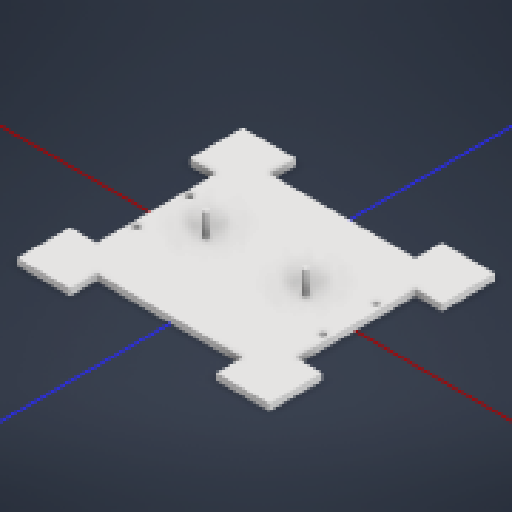
# Autodesk Inventor part: base
Saved by Autodesk Inventor 2025.4 (Build 294407000, 407)
## iProperties
Created: 2026-09-12
Part Number: base
Material: Generic
Document SubType Name: Modeling
Designer: User
Density: 1 g/cm^3
Appearance: Default
Author: User
Autodesk Inventor part; units mm, degrees
ref_plane "YZ Plane" through (0, 0, 0) normal (1, 0, 0) x (0, 1, 0)
ref_plane "XZ Plane" through (0, 0, 0) normal (0, 1, 0) x (-1, 0, 0)
ref_plane "XY Plane" through (0, 0, 0) normal (0, 0, 1) x (1, 0, 0)
sketch "Sketch1" plane through (0, 0, 0) normal (0, 1, 0) x (-1, 0, 0)
  line L0 (15, 13) -> (-15, 13)
  line L1 (-15, 13) -> (-15, -13)
  line L2 (-15, -13) -> (15, -13)
  line L3 (15, -13) -> (15, 13)
  line L4 (15, 13) -> (-15, -13) construction
  line L5 (-15, 13) -> (15, -13) construction
  circle A0 centre (-14, 4) radius 0.5
  circle A1 centre (14, 4) radius 0.5
  circle A2 centre (14, -4) radius 0.5
  circle A3 centre (-14, -4) radius 0.5
  line L6 (-11, 17) -> (-19, 17)
  line L7 (-19, 17) -> (-19, 9)
  line L8 (-19, 9) -> (-11, 9)
  line L9 (-11, 9) -> (-11, 17)
  line L10 (-11, 17) -> (-19, 9) construction
  line L11 (-19, 17) -> (-11, 9) construction
  line L12 (19, 9) -> (11, 9)
  line L13 (11, 9) -> (11, 17)
  line L14 (11, 17) -> (19, 17)
  line L15 (19, 17) -> (19, 9)
  line L16 (19, 9) -> (11, 17) construction
  line L17 (11, 9) -> (19, 17) construction
  line L18 (19, -17) -> (11, -17)
  line L19 (11, -17) -> (11, -9)
  line L20 (11, -9) -> (19, -9)
  line L21 (19, -9) -> (19, -17)
  line L22 (19, -17) -> (11, -9) construction
  line L23 (11, -17) -> (19, -9) construction
  line L24 (-11, -9) -> (-19, -9)
  line L25 (-19, -9) -> (-19, -17)
  line L26 (-19, -17) -> (-11, -17)
  line L27 (-11, -17) -> (-11, -9)
  line L28 (-11, -9) -> (-19, -17) construction
  line L29 (-19, -9) -> (-11, -17) construction
  point P0 (0, 0)
  point P1 (11, 13)
  point P2 (15, 9)
  point P3 (15, -9)
  point P4 (11, -13)
  point P5 (-11, -13)
  point P6 (-15, -9)
  point P7 (-15, 9)
  point P8 (-11, 13)
  dimension "d0" = 30
  dimension "d1" = 26
  dimension "d4" = 1
  dimension "d5" = 9
  dimension "d6" = 1
  dimension "d7" = 1
  dimension "d8" = 1
  dimension "d9" = 1
  dimension "d10" = 1
  dimension "d11" = 9
  dimension "d12" = 1
  dimension "d13" = 9
  dimension "d14" = 9
  dimension "d15" = 1
  dimension "d24" = 8
  dimension "d25" = 8
  dimension "d26" = 8
  dimension "d27" = 8
  dimension "d28" = 8
  dimension "d29" = 8
  dimension "d30" = 8
  dimension "d31" = 8
  constraints: 60 end point, 10 midpoint, 10 parallel, 5 horizontal, 5 perpendicular, 4 centre point
  measures "d0" distance of L2.end L1.end
  measures "d1" distance of L1.end L0.end
  measures "d4" diameter of A0
  measures "d5" distance from line of L0 A0.centre
  measures "d6" distance from line of L1 A0.centre
  measures "d7" diameter of A1
  measures "d8" diameter of A2
  measures "d9" diameter of A3
  measures "d10" distance from line of L1 A3.centre
  measures "d11" distance from line of L2 A3.centre
  measures "d12" distance from line of L3 A2.centre
  measures "d13" distance from line of L2 A2.centre
  measures "d14" distance from line of L0 A1.centre
  measures "d15" distance from line of L3 A1.centre
  measures "d24" distance of L8.end L7.end
  measures "d25" distance of L7.end L6.end
  measures "d26" distance of L13.end L14.end
  measures "d27" distance of L12.end L13.end
  measures "d28" distance of L19.end L20.end
  measures "d29" distance of L18.end L19.end
  measures "d30" distance of L26.end L25.end
  measures "d31" distance of L25.end L24.end
extrude "Extrusion1" add sketch "Sketch1" along normal blind 1
sketch "Sketch3" plane through (0, 1, 0) normal (0, 1, 0) x (1, 0, 0)
  line L0 (15, -9) -> (15, 9) projected
  line L1 (15, 9) -> (19, 9) projected
  line L2 (19, 9) -> (19, 17) projected
  line L3 (19, 17) -> (11, 17) projected
  line L4 (11, 17) -> (11, 13) projected
  line L5 (11, 13) -> (-11, 13) projected
  line L6 (-11, 13) -> (-11, 17) projected
  line L7 (-11, 17) -> (-19, 17) projected
  line L8 (-19, 17) -> (-19, 9) projected
  line L9 (-19, 9) -> (-15, 9) projected
  line L10 (-15, 9) -> (-15, -9) projected
  line L11 (-15, -9) -> (-19, -9) projected
  line L12 (-19, -9) -> (-19, -17) projected
  line L13 (-19, -17) -> (-11, -17) projected
  line L14 (-11, -17) -> (-11, -13) projected
  line L15 (-11, -13) -> (11, -13) projected
  line L16 (11, -13) -> (11, -17) projected
  line L17 (11, -17) -> (19, -17) projected
  line L18 (19, -17) -> (19, -9) projected
  line L19 (19, -9) -> (15, -9) projected
  circle A0 centre (14, -4) radius 0.5 projected
  circle A1 centre (-14, -4) radius 0.5 projected
  circle A2 centre (-14, 4) radius 0.5 projected
  circle A3 centre (14, 4) radius 0.5 projected
  circle A4 centre (-7.5, 0) radius 0.5
  circle A5 centre (7.5, 0) radius 0.5
  point P0 (0, 0)
  dimension "d32" = 1
  dimension "d33" = 1
  dimension "d34" = 7.5
  dimension "d35" = 7.5
  constraints: 2 centre point
  measures "d32" diameter of A4
  measures "d33" diameter of A5
  measures "d34" distance from line of L0 A5.centre
  measures "d35" distance from line of L10 A4.centre
extrude "Extrusion2" add sketch "Sketch3" along normal blind 3.5 contours A4 | A5
sketch "Sketch4" plane through (0, 0, 0) normal (0, -1, 0) x (1, 0, 0)
  line L0 (15, 9) -> (15, -9) projected
  line L1 (19, 9) -> (15, 9) projected
  line L2 (19, 17) -> (19, 9) projected
  line L3 (11, 17) -> (19, 17) projected
  line L4 (11, 13) -> (11, 17) projected
  line L5 (-11, 13) -> (11, 13) projected
  line L6 (-11, 17) -> (-11, 13) projected
  line L7 (-19, 17) -> (-11, 17) projected
  line L8 (-19, 9) -> (-19, 17) projected
  line L9 (-15, 9) -> (-19, 9) projected
  line L10 (-15, -9) -> (-15, 9) projected
  line L11 (-19, -9) -> (-15, -9) projected
  line L12 (-19, -17) -> (-19, -9) projected
  line L13 (-11, -17) -> (-19, -17) projected
  line L14 (-11, -13) -> (-11, -17) projected
  line L15 (11, -13) -> (-11, -13) projected
  line L16 (11, -17) -> (11, -13) projected
  line L17 (19, -17) -> (11, -17) projected
  line L18 (19, -9) -> (19, -17) projected
  line L19 (15, -9) -> (19, -9) projected
  circle A0 centre (14, 4) radius 0.5 projected
  circle A1 centre (-14, 4) radius 0.5 projected
  circle A2 centre (-14, -4) radius 0.5 projected
  circle A3 centre (14, -4) radius 0.5 projected
  circle A4 centre (-7.5, 0) radius 0.5 projected
  circle A5 centre (7.5, 0) radius 0.5 projected
  point P0 (0, 0)
extrude "Extrusion3" cut sketch "Sketch4" against normal blind 0.5 contours A4 | A5
equation "\"d24\" = d25"
equation "\"d26\" = d25"
equation "\"d27\" = d25"
equation "\"d28\" = d25"
equation "\"d29\" = d25"
equation "\"d30\" = d25"
equation "\"d31\" = d25"
body "Solid1"
